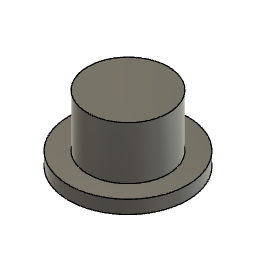
Dual_Diag_Plunger v3 (Autodesk Fusion 360 design; units mm, degrees)
Autodesk Fusion 360 part; units mm, degrees
sketch "Sketch1" plane through (0, 0, 0) normal (0, 1, 0) x (1, 0, 0)
  circle A0 centre (0, 0) radius 4.5
  dimension "d1" = 9
  constraint coincident A0.centre origin
  measures "d1" diameter of A0
extrude "Extrude1" add sketch "Sketch1" along normal blind 1
sketch "Sketch2" plane through (0, 1, 0) normal (0, 1, 0) x (-1, 0, 0)
  circle A0 centre (0, 0) radius 4.5
  circle A1 centre (0, 0) radius 3.048
  dimension "d4" = 6.096
  constraint coincident A0.centre A1.centre
  measures "d4" diameter of A1
extrude "Extrude2" add sketch "Sketch2" along normal blind 4 contours A1
sketch "Sketch3" plane through (0, 0, 0) normal (0, -1, 0) x (1, 0, 0)
  circle A0 centre (0, 0) radius 4.5
  circle A1 centre (0, 0) radius 1.778
  dimension "d7" = 3.556
  constraint concentric A0 A1
  measures "d7" diameter of A1
extrude "Extrude3" cut sketch "Sketch3" against normal blind 4 contours A1
